sharps (Autodesk Fusion 360 design; units mm, degrees)
Autodesk Fusion 360 part; units mm, degrees
(part 1 of 2)
sketch "Sketch1" plane through (0, 0, 0) normal (0, 1, 0) x (1, 0, 0)
  line L0 (0, 0) -> (-92, 0)
  line L1 (-92, 0) -> (-92, -56)
  line L2 (-92, -56) -> (0, -56)
  line L3 (0, -56) -> (0, 0)
  dimension "d1" = 92
  dimension "d2" = 56
  constraint horizontal L0
  constraint vertical L1
  constraint horizontal L2
  constraint vertical L3
  constraint coincident L0.start L3.end
  measures "d1" distance of L1.end L2.end
  measures "d2" distance of L0.start L2.end
extrude "Extrude1" add sketch "Sketch1" along normal blind 65
shell "Shell1" thickness 3.5 removed faces 1 at (-30.6667, 65, 18.6667)
fillet "Fillet1" radius 5 8 edges at (0, 32.5, 0) (0, 32.5, 56) (-92, 32.5, 56) (-92, 32.5, 0) (-3.5, 34.25, 3.5) (-3.5, 34.25, 52.5) (-88.5, 34.25, 52.5) (-88.5, 34.25, 3.5)
extrude "Extrude2" add 1 faces at (-32.3333, 0, 37.3333) along direction (0, 1, 0) blind 3.5 from surface at 65
sketch "Sketch2" plane through (0, 68.5, 0) normal (0, 1, 0) x (-1, 0, 0)
  line L0 (5, 0) -> (87, 0)
  arc A0 (87, 0) -> (92, 5) centre (87, 5) ccw
  line L1 (92, 5) -> (92, 51)
  arc A1 (92, 51) -> (87, 56) centre (87, 51) ccw
  line L2 (87, 56) -> (5, 56)
  arc A2 (5, 56) -> (0, 51) centre (5, 51) ccw
  line L3 (0, 51) -> (0, 5)
  arc A3 (0, 5) -> (5, 0) centre (5, 5) ccw
  line L4 (85, 26.75) -> (7, 26.75)
  line L5 (7, 26.75) -> (7, 29.25)
  line L6 (7, 29.25) -> (85, 29.25)
  line L7 (85, 29.25) -> (85, 26.75)
  dimension "d11" = 26.75
  dimension "d12" = 26.75
  dimension "d13" = 7
  dimension "d14" = 7
  constraint horizontal L4
  constraint vertical L5
  constraint horizontal L6
  constraint vertical L7
  measures "d11" distance of L0 L4
  measures "d12" distance of L2 L6
  measures "d13" distance of L3 L5
  measures "d14" distance of L1 L7
extrude "Extrude3" cut sketch "Sketch2" against normal blind 40 contours L4 L5 L6 L7
chamfer "Chamfer1" distance 2 angle 45 2 edges at (-46, 68.5, 26.75) (-46, 68.5, 29.25)
ref_plane "WorkPlane1" through (-46, 42.5, 28) normal (0, 1, 0) x (0, 0, 1)
sketch "Sketch3" plane through (0, 65, 0) normal (0, -1, 0) x (1, 0, 0)
  line L0 (-7, 29.25) -> (-7, 26.75)
  line L1 (-7, 26.75) -> (-85, 26.75)
  line L2 (-85, 26.75) -> (-85, 29.25)
  line L3 (-85, 29.25) -> (-7, 29.25)
  arc A0 (-83.5, 52.5) -> (-88.5, 47.5) centre (-83.5, 47.5) ccw
  line L4 (-88.5, 47.5) -> (-88.5, 8.5)
  arc A1 (-88.5, 8.5) -> (-83.5, 3.5) centre (-83.5, 8.5) ccw
  line L5 (-83.5, 3.5) -> (-8.5, 3.5)
  arc A2 (-8.5, 3.5) -> (-3.5, 8.5) centre (-8.5, 8.5) ccw
  line L6 (-3.5, 8.5) -> (-3.5, 47.5)
  arc A3 (-3.5, 47.5) -> (-8.5, 52.5) centre (-8.5, 47.5) ccw
  line L7 (-8.5, 52.5) -> (-83.5, 52.5)
  line L8 (-3.5, 37.1108) -> (-18.952, 52.5)
  line L9 (-73, 52.5) -> (-88.5, 33.8548)
  line L10 (-88.5, 16) -> (-69.7967, 3.5)
  line L11 (-23, 3.5) -> (-3.5, 18.2423)
  line L12 (-3.5, 28) -> (-46, 3.5)
  line L13 (-88.5, 28) -> (-46, 3.5)
  line L14 (-88.5, 28) -> (-46, 52.5)
  line L15 (-3.5, 28) -> (-46, 52.5)
  line L16 (-24.75, 40.25) -> (-67.25, 40.25)
  line L17 (-67.25, 15.75) -> (-24.75, 15.75)
  line L18 (-85, 26.75) -> (-85, 25.9)
  line L19 (-85, 25.9) -> (-85, 30.1)
  line L20 (-7, 26.75) -> (-7, 25.8)
  line L21 (-7, 25.8) -> (-7, 30.2)
  line L22 (-85, 29.25) -> (-46, 40.25)
  line L23 (-7, 29.25) -> (-46, 40.25)
  line L24 (-85, 26.75) -> (-46, 15.75)
  line L25 (-46, 15.75) -> (-7, 26.75)
  line L26 (-26.5, 21.25) -> (-65.5, 21.25)
  line L27 (-65.5, 34.75) -> (-26.5, 34.75)
  constraint coincident L6 L8.start
  constraint coincident L7 L8.end
  constraint coincident L7 L9.start
  constraint coincident L4 L9.end
  constraint coincident L4 L10.start
  constraint coincident L5 L10.end
  constraint coincident L5 L11.start
  constraint coincident L6 L11.end
  constraint midpoint L6 L12.start
  constraint coincident L5 L12.end
  constraint midpoint L4 L13.start
  constraint midpoint L7 L14.end
  constraint midpoint L5 L12.end
  constraint midpoint L15 L16.start
  constraint midpoint L14 L16.end
  constraint midpoint L13 L17.start
  constraint midpoint L12 L17.end
  constraint coincident L1.end L2.start
  constraint perpendicular L1 L18
  constraint parallel L2 L19
  constraint coincident L0.end L1.start
  constraint perpendicular L1 L20
  constraint perpendicular L3 L21
  constraint coincident L2.end L3.start
  constraint midpoint L16 L22.end
  constraint coincident L0.start L3.end
  constraint midpoint L17 L24.end
  constraint midpoint L25 L26.start
  constraint midpoint L24 L26.end
  constraint midpoint L22 L27.start
  constraint midpoint L23 L27.end
sketch "Sketch4" plane through (0, 68.5, 0) normal (0, 1, 0) x (-1, 0, 0)
  line L0 (85, 31.25) -> (85, 24.75)
  line L1 (85, 24.75) -> (7, 24.75)
  line L2 (7, 24.75) -> (7, 31.25)
  line L3 (7, 31.25) -> (85, 31.25)
  line L4 (5, 0) -> (87, 0)
  arc A0 (87, 0) -> (92, 5) centre (87, 5) ccw
  line L5 (92, 5) -> (92, 51)
  arc A1 (92, 51) -> (87, 56) centre (87, 51) ccw
  line L6 (87, 56) -> (5, 56)
  arc A2 (5, 56) -> (0, 51) centre (5, 51) ccw
  line L7 (0, 51) -> (0, 5)
  arc A3 (0, 5) -> (5, 0) centre (5, 5) ccw
  spline S0 degree 3 poles (69.4034, 34.4959) (69.5108, 34.5366) (69.6516, 34.6404) (69.8145, 34.7996) knots 0 0 0 0 1 1 1 1
  spline S1 degree 3 poles (69.8145, 34.7996) (70.0442, 35.0293) (70.3331, 35.522) (74.9596, 43.5267) knots 0 0 0 0 1 1 1 1
  spline S2 degree 3 poles (74.9596, 43.5267) (77.6563, 48.1902) (79.901, 52.0981) (79.9491, 52.2129) knots 0 0 0 0 1 1 1 1
  spline S3 degree 3 poles (79.9491, 52.2129) (80.0492, 52.4574) (80.0603, 52.8241) (79.9751, 53.0723) knots 0 0 0 0 1 1 1 1
  spline S4 degree 3 poles (79.9751, 53.0723) (79.901, 53.2945) (79.7158, 53.5057) (79.4824, 53.6316) knots 0 0 0 0 1 1 1 1
  spline S5 degree 3 poles (79.4824, 53.6316) (79.0787, 53.8539) (79.6861, 53.8428) (68.9552, 53.8428) knots 0 0 0 0 1 1 1 1
  spline S6 degree 3 poles (68.9552, 53.8428) (62.4988, 53.8428) (59.0465, 53.8316) (58.9206, 53.8057) knots 0 0 0 0 1 1 1 1
  spline S7 degree 3 poles (58.9206, 53.8057) (58.4835, 53.7242) (58.139, 53.476) (57.9797, 53.139) knots 0 0 0 0 1 1 1 1
  spline S8 degree 3 poles (57.9797, 53.139) (57.8797, 52.9204) (57.8797, 52.5278) (57.9834, 52.2685) knots 0 0 0 0 1 1 1 1
  spline S9 degree 3 poles (57.9834, 52.2685) (58.0205, 52.1648) (60.2874, 48.2384) (63.0174, 43.5452) knots 0 0 0 0 1 1 1 1
  spline S10 degree 3 poles (63.0174, 43.5452) (68.4477, 34.1959) (68.1514, 34.6774) (68.5996, 34.5107) knots 0 0 0 0 1 1 1 1
  spline S11 degree 3 poles (68.5996, 34.5107) (68.8515, 34.4181) (69.1626, 34.4144) (69.4034, 34.4959) knots 0 0 0 0 1 1 1 1
  spline S12 degree 3 poles (68.6144, 34.6885) (68.5292, 34.7256) (68.3847, 34.833) (68.2921, 34.9256) knots 0 0 0 0 1 1 1 1
  spline S13 degree 3 poles (68.2921, 34.9256) (68.1736, 35.0515) (66.7697, 37.437) (63.1693, 43.6267) knots 0 0 0 0 1 1 1 1
  spline S14 degree 3 poles (63.1693, 43.6267) (60.443, 48.3198) (58.1761, 52.2463) (58.139, 52.3574) knots 0 0 0 0 1 1 1 1
  spline S15 degree 3 poles (58.139, 52.3574) (57.9538, 52.8908) (58.1909, 53.3909) (58.7169, 53.5724) knots 0 0 0 0 1 1 1 1
  spline S16 degree 3 poles (58.7169, 53.5724) (58.891, 53.6353) (59.4577, 53.639) (68.9589, 53.639) knots 0 0 0 0 1 1 1 1
  spline S17 degree 3 poles (68.9589, 53.639) (78.5119, 53.639) (79.0268, 53.6353) (79.2046, 53.5724) knots 0 0 0 0 1 1 1 1
  spline S18 degree 3 poles (79.2046, 53.5724) (79.438, 53.4909) (79.6787, 53.2908) (79.7825, 53.0871) knots 0 0 0 0 1 1 1 1
  spline S19 degree 3 poles (79.7825, 53.0871) (79.8825, 52.8982) (79.8899, 52.4907) (79.7936, 52.2722) knots 0 0 0 0 1 1 1 1
  spline S20 degree 3 poles (79.7936, 52.2722) (79.6824, 52.0129) (69.9183, 35.1589) (69.7849, 34.9997) knots 0 0 0 0 1 1 1 1
  spline S21 degree 3 poles (69.7849, 34.9997) (69.6479, 34.8293) (69.396, 34.6626) (69.2071, 34.6144) knots 0 0 0 0 1 1 1 1
  spline S22 degree 3 poles (69.2071, 34.6144) (69.0515, 34.5774) (68.8033, 34.607) (68.6144, 34.6885) knots 0 0 0 0 1 1 1 1
  spline S23 degree 3 poles (69.2367, 35.2071) (69.3182, 35.2441) (69.4219, 35.3145) (69.4664, 35.3627) knots 0 0 0 0 1 1 1 1
  spline S24 degree 3 poles (69.4664, 35.3627) (69.6034, 35.5145) (79.2528, 52.2166) (79.2787, 52.3463) knots 0 0 0 0 1 1 1 1
  spline S25 degree 3 poles (79.2787, 52.3463) (79.3305, 52.6315) (79.2157, 52.8575) (78.949, 53.0019) knots 0 0 0 0 1 1 1 1
  line L8 (78.949, 53.0019) -> (78.7934, 53.0834)
  line L9 (78.7934, 53.0834) -> (68.9996, 53.0945)
  line L10 (68.9996, 53.0945) -> (59.2058, 53.1019)
  line L11 (59.2058, 53.1019) -> (59.0095, 53.013)
  spline S26 degree 3 poles (59.0095, 53.013) (58.8798, 52.9538) (58.7835, 52.8797) (58.7354, 52.7982) knots 0 0 0 0 1 1 1 1
  spline S27 degree 3 poles (58.7354, 52.7982) (58.6502, 52.6537) (58.6391, 52.413) (58.7132, 52.2389) knots 0 0 0 0 1 1 1 1
  spline S28 degree 3 poles (58.7132, 52.2389) (58.7391, 52.1722) (60.932, 48.3865) (63.5841, 43.823) knots 0 0 0 0 1 1 1 1
  spline S29 degree 3 poles (63.5841, 43.823) (66.7808, 38.326) (68.4588, 35.4738) (68.5588, 35.3738) knots 0 0 0 0 1 1 1 1
  spline S30 degree 3 poles (68.5588, 35.3738) (68.6885, 35.2367) (68.8959, 35.1367) (69.0367, 35.1367) knots 0 0 0 0 1 1 1 1
  spline S31 degree 3 poles (69.0367, 35.1367) (69.0663, 35.1367) (69.1552, 35.1701) (69.2367, 35.2071) knots 0 0 0 0 1 1 1 1
  spline S32 degree 3 poles (64.2398, 44.3156) (61.6802, 48.6643) (59.5873, 52.224) (59.5873, 52.2352) knots 0 0 0 0 1 1 1 1
  spline S33 degree 3 poles (59.5873, 52.2352) (59.5873, 52.2426) (63.8027, 52.25) (68.9589, 52.25) knots 0 0 0 0 1 1 1 1
  spline S34 degree 3 poles (68.9589, 52.25) (74.1151, 52.25) (78.3304, 52.2389) (78.3304, 52.2277) knots 0 0 0 0 1 1 1 1
  spline S35 degree 3 poles (78.3304, 52.2277) (78.3304, 52.1685) (68.9404, 36.3628) (68.9181, 36.3887) knots 0 0 0 0 1 1 1 1
  spline S36 degree 3 poles (68.9181, 36.3887) (68.907, 36.4035) (66.7994, 39.9707) (64.2398, 44.3156) knots 0 0 0 0 1 1 1 1
  spline S37 degree 3 poles (70.0627, 42.6562) (70.9517, 42.7969) (71.4777, 42.8932) (71.537, 42.934) knots 0 0 0 0 1 1 1 1
  spline S38 degree 3 poles (71.537, 42.934) (71.5851, 42.9673) (71.674, 43.0785) (71.7296, 43.1822) knots 0 0 0 0 1 1 1 1
  spline S39 degree 3 poles (71.7296, 43.1822) (71.7852, 43.2896) (71.8741, 43.4229) (71.9296, 43.4785) knots 0 0 0 0 1 1 1 1
  spline S40 degree 3 poles (71.9296, 43.4785) (72.0222, 43.5785) (72.0445, 43.5822) (72.363, 43.5822) knots 0 0 0 0 1 1 1 1
  line L12 (72.363, 43.5822) -> (72.7001, 43.5822)
  line L13 (72.7001, 43.5822) -> (72.7001, 44.6194)
  line L14 (72.7001, 44.6194) -> (72.7001, 45.6566)
  line L15 (72.7001, 45.6566) -> (72.3371, 45.6566)
  spline S41 degree 3 poles (72.3371, 45.6566) (71.9333, 45.6566) (71.9185, 45.664) (71.7407, 45.9603) knots 0 0 0 0 1 1 1 1
  spline S42 degree 3 poles (71.7407, 45.9603) (71.6889, 46.0455) (71.6148, 46.1122) (71.5407, 46.1344) knots 0 0 0 0 1 1 1 1
  spline S43 degree 3 poles (71.5407, 46.1344) (71.337, 46.2011) (68.2921, 46.2048) (67.818, 46.1381) knots 0 0 0 0 1 1 1 1
  spline S44 degree 3 poles (67.818, 46.1381) (67.6698, 46.1196) (67.2031, 46.1011) (66.7882, 46.1011) knots 0 0 0 0 1 1 1 1
  spline S45 degree 3 poles (66.7882, 46.1011) (66.3549, 46.1011) (65.9993, 46.0862) (65.9585, 46.064) knots 0 0 0 0 1 1 1 1
  spline S46 degree 3 poles (65.9585, 46.064) (65.8511, 46.0084) (65.7955, 45.7936) (65.8474, 45.6417) knots 0 0 0 0 1 1 1 1
  spline S47 degree 3 poles (65.8474, 45.6417) (65.9178, 45.4232) (65.9178, 45.4232) (66.7216, 45.4676) knots 0 0 0 0 1 1 1 1
  spline S48 degree 3 poles (66.7216, 45.4676) (67.3846, 45.5047) (67.5217, 45.501) (67.4735, 45.4565) knots 0 0 0 0 1 1 1 1
  spline S49 degree 3 poles (67.4735, 45.4565) (67.4661, 45.4491) (67.0031, 45.4269) (66.4438, 45.4047) knots 0 0 0 0 1 1 1 1
  spline S50 degree 3 poles (66.4438, 45.4047) (65.4584, 45.3713) (65.4251, 45.3676) (65.3584, 45.2861) knots 0 0 0 0 1 1 1 1
  spline S51 degree 3 poles (65.3584, 45.2861) (65.2732, 45.1824) (65.2695, 44.9268) (65.351, 44.8083) knots 0 0 0 0 1 1 1 1
  line L16 (65.351, 44.8083) -> (65.414, 44.7194)
  line L17 (65.414, 44.7194) -> (66.3808, 44.7416)
  spline S52 degree 3 poles (66.3808, 44.7416) (66.9623, 44.7527) (67.2068, 44.749) (66.9957, 44.7305) knots 0 0 0 0 1 1 1 1
  spline S53 degree 3 poles (66.9957, 44.7305) (66.8031, 44.7157) (66.2622, 44.7009) (65.7992, 44.6972) knots 0 0 0 0 1 1 1 1
  line L18 (65.7992, 44.6972) -> (64.9547, 44.6935)
  line L19 (64.9547, 44.6935) -> (64.8658, 44.6009)
  spline S54 degree 3 poles (64.8658, 44.6009) (64.7547, 44.4934) (64.7398, 44.2416) (64.8361, 44.1045) knots 0 0 0 0 1 1 1 1
  line L20 (64.8361, 44.1045) -> (64.8954, 44.0156)
  line L21 (64.8954, 44.0156) -> (66.04, 44.0415)
  spline S55 degree 3 poles (66.04, 44.0415) (66.7253, 44.0564) (67.1809, 44.0526) (67.1809, 44.0341) knots 0 0 0 0 1 1 1 1
  spline S56 degree 3 poles (67.1809, 44.0341) (67.1809, 43.9934) (66.8549, 43.9637) (66.0363, 43.9304) knots 0 0 0 0 1 1 1 1
  spline S57 degree 3 poles (66.0363, 43.9304) (65.3658, 43.9008) (65.3288, 43.8823) (65.3288, 43.5896) knots 0 0 0 0 1 1 1 1
  spline S58 degree 3 poles (65.3288, 43.5896) (65.3288, 43.4933) (65.3547, 43.3785) (65.3807, 43.3377) knots 0 0 0 0 1 1 1 1
  spline S59 degree 3 poles (65.3807, 43.3377) (65.4362, 43.2637) (65.4621, 43.26) (67.0586, 43.2563) knots 0 0 0 0 1 1 1 1
  spline S60 degree 3 poles (67.0586, 43.2563) (67.9921, 43.2525) (68.8589, 43.2674) (69.0996, 43.2896) knots 0 0 0 0 1 1 1 1
  spline S61 degree 3 poles (69.0996, 43.2896) (69.3293, 43.3118) (69.5256, 43.3229) (69.5367, 43.3155) knots 0 0 0 0 1 1 1 1
  spline S62 degree 3 poles (69.5367, 43.3155) (69.5441, 43.3044) (69.3886, 43.2525) (69.1922, 43.1933) knots 0 0 0 0 1 1 1 1
  spline S63 degree 3 poles (69.1922, 43.1933) (68.7774, 43.0785) (68.67, 43.0007) (68.5514, 42.7229) knots 0 0 0 0 1 1 1 1
  spline S64 degree 3 poles (68.5514, 42.7229) (68.4625, 42.5117) (68.4736, 42.4339) (68.5959, 42.4376) knots 0 0 0 0 1 1 1 1
  spline S65 degree 3 poles (68.5959, 42.4376) (68.644, 42.4413) (69.3034, 42.5376) (70.0627, 42.6562) knots 0 0 0 0 1 1 1 1
  spline S66 degree 3 poles (68.6625, 43.4229) (68.6588, 43.4415) (68.7885, 43.8971) (68.9478, 44.4416) knots 0 0 0 0 1 1 1 1
  line L22 (68.9478, 44.4416) -> (69.2367, 45.4306)
  line L23 (69.2367, 45.4306) -> (69.2478, 44.4638)
  spline S67 degree 3 poles (69.2478, 44.4638) (69.2515, 43.9304) (69.2478, 43.4896) (69.2367, 43.4785) knots 0 0 0 0 1 1 1 1
  spline S68 degree 3 poles (69.2367, 43.4785) (69.2256, 43.4674) (69.107, 43.4452) (68.9663, 43.4341) knots 0 0 0 0 1 1 1 1
  spline S69 degree 3 poles (68.9663, 43.4341) (68.8292, 43.4192) (68.707, 43.4044) (68.6885, 43.4007) knots 0 0 0 0 1 1 1 1
  spline S70 degree 3 poles (68.6885, 43.4007) (68.6737, 43.4007) (68.6625, 43.4081) (68.6625, 43.4229) knots 0 0 0 0 1 1 1 1
  spline S71 degree 3 poles (67.8476, 43.4303) (67.8476, 43.4452) (67.9884, 43.9008) (68.1625, 44.4379) knots 0 0 0 0 1 1 1 1
  line L24 (68.1625, 44.4379) -> (68.4736, 45.4158)
  line L25 (68.4736, 45.4158) -> (68.4736, 44.9342)
  spline S72 degree 3 poles (68.4736, 44.9342) (68.4773, 44.6675) (68.4662, 44.2156) (68.4514, 43.923) knots 0 0 0 0 1 1 1 1
  line L26 (68.4514, 43.923) -> (68.4292, 43.397)
  line L27 (68.4292, 43.397) -> (68.1366, 43.397)
  spline S73 degree 3 poles (68.1366, 43.397) (67.9773, 43.397) (67.8476, 43.4118) (67.8476, 43.4303) knots 0 0 0 0 1 1 1 1
  spline S74 degree 3 poles (67.3253, 43.4341) (67.2253, 43.4341) (67.2327, 43.6637) (67.3476, 44.2045) knots 0 0 0 0 1 1 1 1
  spline S75 degree 3 poles (67.3476, 44.2045) (67.4735, 44.7898) (67.7735, 45.927) (67.8143, 45.9677) knots 0 0 0 0 1 1 1 1
  spline S76 degree 3 poles (67.8143, 45.9677) (67.8587, 46.0159) (67.8624, 46.0529) (67.755, 44.7676) knots 0 0 0 0 1 1 1 1
  spline S77 degree 3 poles (67.755, 44.7676) (67.6328, 43.2933) (67.6476, 43.3822) (67.5068, 43.4118) knots 0 0 0 0 1 1 1 1
  spline S78 degree 3 poles (67.5068, 43.4118) (67.4439, 43.4229) (67.3624, 43.4341) (67.3253, 43.4341) knots 0 0 0 0 1 1 1 1
  line L28 (69.4404, 44.8972) -> (69.4404, 46.027)
  line L29 (69.4404, 46.027) -> (69.7368, 46.027)
  spline S79 degree 3 poles (69.7368, 46.027) (69.9664, 46.027) (70.0331, 46.0159) (70.0331, 45.9751) knots 0 0 0 0 1 1 1 1
  spline S80 degree 3 poles (70.0331, 45.9751) (70.0331, 45.7269) (69.5219, 43.7674) (69.4589, 43.7674) knots 0 0 0 0 1 1 1 1
  spline S81 degree 3 poles (69.4589, 43.7674) (69.4478, 43.7674) (69.4404, 44.2749) (69.4404, 44.8972) knots 0 0 0 0 1 1 1 1
  line L30 (68.6514, 45.038) -> (68.6737, 46.027)
  line L31 (68.6737, 46.027) -> (68.9478, 46.027)
  spline S82 degree 3 poles (68.9478, 46.027) (69.0959, 46.027) (69.2182, 46.0159) (69.2182, 45.9973) knots 0 0 0 0 1 1 1 1
  spline S83 degree 3 poles (69.2182, 45.9973) (69.2219, 45.9529) (68.6477, 44.0304) (68.6366, 44.0415) knots 0 0 0 0 1 1 1 1
  spline S84 degree 3 poles (68.6366, 44.0415) (68.6292, 44.0452) (68.6366, 44.4971) (68.6514, 45.038) knots 0 0 0 0 1 1 1 1
  spline S85 degree 3 poles (67.9513, 45.1528) (68.0032, 45.7455) (68.0365, 45.9677) (68.0736, 45.9936) knots 0 0 0 0 1 1 1 1
  spline S86 degree 3 poles (68.0736, 45.9936) (68.1588, 46.0455) (68.4885, 46.0344) (68.4699, 45.9788) knots 0 0 0 0 1 1 1 1
  spline S87 degree 3 poles (68.4699, 45.9788) (68.4588, 45.9566) (68.3292, 45.5417) (68.1773, 45.0565) knots 0 0 0 0 1 1 1 1
  spline S88 degree 3 poles (68.1773, 45.0565) (68.0254, 44.5749) (67.8995, 44.2156) (67.8921, 44.2601) knots 0 0 0 0 1 1 1 1
  spline S89 degree 3 poles (67.8921, 44.2601) (67.8884, 44.3045) (67.9143, 44.7046) (67.9513, 45.1528) knots 0 0 0 0 1 1 1 1
  line L32 (69.3071, 47.9568) -> (70.1442, 49.031)
  line L33 (70.1442, 49.031) -> (70.1442, 50.4942)
  line L34 (70.1442, 50.4942) -> (70.1442, 51.9536)
  line L35 (70.1442, 51.9536) -> (69.2923, 51.9536)
  line L36 (69.2923, 51.9536) -> (68.4403, 51.9536)
  line L37 (68.4403, 51.9536) -> (68.4403, 49.4163)
  spline S90 degree 3 poles (68.4403, 49.4163) (68.4403, 48.0198) (68.4477, 46.8789) (68.4551, 46.8789) knots 0 0 0 0 1 1 1 1
  spline S91 degree 3 poles (68.4551, 46.8789) (68.4662, 46.8789) (68.8478, 47.3642) (69.3071, 47.9568) knots 0 0 0 0 1 1 1 1
  spline S92 degree 3 poles (57.9797, 53.139) (57.8797, 52.9204) (57.8797, 52.5278) (57.9834, 52.2685) knots 0 0 0 0 1 1 1 1
  line L38 (69.2923, 51.9536) -> (68.4403, 51.9536)
  spline S93 degree 3 poles (64.2398, 44.3156) (61.6802, 48.6643) (59.5873, 52.224) (59.5873, 52.2352) knots 0 0 0 0 1 1 1 1
  line L39 (68.4403, 51.9536) -> (68.4403, 49.4163)
  spline S94 degree 3 poles (57.9834, 52.2685) (58.0205, 52.1648) (60.2874, 48.2384) (63.0174, 43.5452) knots 0 0 0 0 1 1 1 1
  spline S95 degree 3 poles (59.0095, 53.013) (58.8798, 52.9538) (58.7835, 52.8797) (58.7354, 52.7982) knots 0 0 0 0 1 1 1 1
  spline S96 degree 3 poles (58.139, 52.3574) (57.9538, 52.8908) (58.1909, 53.3909) (58.7169, 53.5724) knots 0 0 0 0 1 1 1 1
  spline S97 degree 3 poles (69.5367, 43.3155) (69.5441, 43.3044) (69.3886, 43.2525) (69.1922, 43.1933) knots 0 0 0 0 1 1 1 1
  spline S98 degree 3 poles (67.4735, 45.4565) (67.4661, 45.4491) (67.0031, 45.4269) (66.4438, 45.4047) knots 0 0 0 0 1 1 1 1
  spline S99 degree 3 poles (67.8921, 44.2601) (67.8884, 44.3045) (67.9143, 44.7046) (67.9513, 45.1528) knots 0 0 0 0 1 1 1 1
  spline S100 degree 3 poles (68.5959, 42.4376) (68.644, 42.4413) (69.3034, 42.5376) (70.0627, 42.6562) knots 0 0 0 0 1 1 1 1
  line L40 (65.414, 44.7194) -> (66.3808, 44.7416)
  line L41 (69.3071, 47.9568) -> (70.1442, 49.031)
  spline S101 degree 3 poles (65.8474, 45.6417) (65.9178, 45.4232) (65.9178, 45.4232) (66.7216, 45.4676) knots 0 0 0 0 1 1 1 1
  line L42 (70.1442, 49.031) -> (70.1442, 50.4942)
  spline S102 degree 3 poles (67.1809, 44.0341) (67.1809, 43.9934) (66.8549, 43.9637) (66.0363, 43.9304) knots 0 0 0 0 1 1 1 1
  line L43 (70.1442, 51.9536) -> (69.2923, 51.9536)
  spline S103 degree 3 poles (70.0627, 42.6562) (70.9517, 42.7969) (71.4777, 42.8932) (71.537, 42.934) knots 0 0 0 0 1 1 1 1
  spline S104 degree 3 poles (64.8658, 44.6009) (64.7547, 44.4934) (64.7398, 44.2416) (64.8361, 44.1045) knots 0 0 0 0 1 1 1 1
  line L44 (72.7001, 43.5822) -> (72.7001, 44.6194)
  spline S105 degree 3 poles (66.9957, 44.7305) (66.8031, 44.7157) (66.2622, 44.7009) (65.7992, 44.6972) knots 0 0 0 0 1 1 1 1
  line L45 (68.4292, 43.397) -> (68.1366, 43.397)
  spline S106 degree 3 poles (69.2182, 45.9973) (69.2219, 45.9529) (68.6477, 44.0304) (68.6366, 44.0415) knots 0 0 0 0 1 1 1 1
  spline S107 degree 3 poles (67.8476, 43.4303) (67.8476, 43.4452) (67.9884, 43.9008) (68.1625, 44.4379) knots 0 0 0 0 1 1 1 1
  line L46 (68.4736, 45.4158) -> (68.4736, 44.9342)
  spline S108 degree 3 poles (66.04, 44.0415) (66.7253, 44.0564) (67.1809, 44.0526) (67.1809, 44.0341) knots 0 0 0 0 1 1 1 1
  spline S109 degree 3 poles (69.4589, 43.7674) (69.4478, 43.7674) (69.4404, 44.2749) (69.4404, 44.8972) knots 0 0 0 0 1 1 1 1
  spline S110 degree 3 poles (68.5514, 42.7229) (68.4625, 42.5117) (68.4736, 42.4339) (68.5959, 42.4376) knots 0 0 0 0 1 1 1 1
  spline S111 degree 3 poles (68.4699, 45.9788) (68.4588, 45.9566) (68.3292, 45.5417) (68.1773, 45.0565) knots 0 0 0 0 1 1 1 1
  spline S112 degree 3 poles (67.3476, 44.2045) (67.4735, 44.7898) (67.7735, 45.927) (67.8143, 45.9677) knots 0 0 0 0 1 1 1 1
  line L47 (64.9547, 44.6935) -> (64.8658, 44.6009)
  spline S113 degree 3 poles (71.9296, 43.4785) (72.0222, 43.5785) (72.0445, 43.5822) (72.363, 43.5822) knots 0 0 0 0 1 1 1 1
  spline S114 degree 3 poles (65.3584, 45.2861) (65.2732, 45.1824) (65.2695, 44.9268) (65.351, 44.8083) knots 0 0 0 0 1 1 1 1
  line L48 (64.8361, 44.1045) -> (64.8954, 44.0156)
  spline S115 degree 3 poles (69.1922, 43.1933) (68.7774, 43.0785) (68.67, 43.0007) (68.5514, 42.7229) knots 0 0 0 0 1 1 1 1
  spline S116 degree 3 poles (68.4403, 49.4163) (68.4403, 48.0198) (68.4477, 46.8789) (68.4551, 46.8789) knots 0 0 0 0 1 1 1 1
  line L49 (59.2058, 53.1019) -> (59.0095, 53.013)
  spline S117 degree 3 poles (68.9589, 52.25) (74.1151, 52.25) (78.3304, 52.2389) (78.3304, 52.2277) knots 0 0 0 0 1 1 1 1
  spline S118 degree 3 poles (68.4551, 46.8789) (68.4662, 46.8789) (68.8478, 47.3642) (69.3071, 47.9568) knots 0 0 0 0 1 1 1 1
  line L50 (68.9996, 53.0945) -> (59.2058, 53.1019)
  spline S119 degree 3 poles (68.1366, 43.397) (67.9773, 43.397) (67.8476, 43.4118) (67.8476, 43.4303) knots 0 0 0 0 1 1 1 1
  spline S120 degree 3 poles (59.5873, 52.2352) (59.5873, 52.2426) (63.8027, 52.25) (68.9589, 52.25) knots 0 0 0 0 1 1 1 1
  spline S121 degree 3 poles (67.0586, 43.2563) (67.9921, 43.2525) (68.8589, 43.2674) (69.0996, 43.2896) knots 0 0 0 0 1 1 1 1
  spline S122 degree 3 poles (65.3288, 43.5896) (65.3288, 43.4933) (65.3547, 43.3785) (65.3807, 43.3377) knots 0 0 0 0 1 1 1 1
  line L51 (68.4514, 43.923) -> (68.4292, 43.397)
  spline S123 degree 3 poles (71.537, 42.934) (71.5851, 42.9673) (71.674, 43.0785) (71.7296, 43.1822) knots 0 0 0 0 1 1 1 1
  line L52 (78.949, 53.0019) -> (78.7934, 53.0834)
  spline S124 degree 3 poles (69.0367, 35.1367) (69.0663, 35.1367) (69.1552, 35.1701) (69.2367, 35.2071) knots 0 0 0 0 1 1 1 1
  spline S125 degree 3 poles (69.2367, 35.2071) (69.3182, 35.2441) (69.4219, 35.3145) (69.4664, 35.3627) knots 0 0 0 0 1 1 1 1
  spline S126 degree 3 poles (68.9552, 53.8428) (62.4988, 53.8428) (59.0465, 53.8316) (58.9206, 53.8057) knots 0 0 0 0 1 1 1 1
  spline S127 degree 3 poles (69.4664, 35.3627) (69.6034, 35.5145) (79.2528, 52.2166) (79.2787, 52.3463) knots 0 0 0 0 1 1 1 1
  spline S128 degree 3 poles (79.7936, 52.2722) (79.6824, 52.0129) (69.9183, 35.1589) (69.7849, 34.9997) knots 0 0 0 0 1 1 1 1
  spline S129 degree 3 poles (78.3304, 52.2277) (78.3304, 52.1685) (68.9404, 36.3628) (68.9181, 36.3887) knots 0 0 0 0 1 1 1 1
  spline S130 degree 3 poles (69.8145, 34.7996) (70.0442, 35.0293) (70.3331, 35.522) (74.9596, 43.5267) knots 0 0 0 0 1 1 1 1
  spline S131 degree 3 poles (68.9589, 53.639) (78.5119, 53.639) (79.0268, 53.6353) (79.2046, 53.5724) knots 0 0 0 0 1 1 1 1
  spline S132 degree 3 poles (79.4824, 53.6316) (79.0787, 53.8539) (79.6861, 53.8428) (68.9552, 53.8428) knots 0 0 0 0 1 1 1 1
  spline S133 degree 3 poles (63.5841, 43.823) (66.7808, 38.326) (68.4588, 35.4738) (68.5588, 35.3738) knots 0 0 0 0 1 1 1 1
  spline S134 degree 3 poles (58.7169, 53.5724) (58.891, 53.6353) (59.4577, 53.639) (68.9589, 53.639) knots 0 0 0 0 1 1 1 1
  spline S135 degree 3 poles (68.6144, 34.6885) (68.5292, 34.7256) (68.3847, 34.833) (68.2921, 34.9256) knots 0 0 0 0 1 1 1 1
  spline S136 degree 3 poles (68.9181, 36.3887) (68.907, 36.4035) (66.7994, 39.9707) (64.2398, 44.3156) knots 0 0 0 0 1 1 1 1
  spline S137 degree 3 poles (69.2071, 34.6144) (69.0515, 34.5774) (68.8033, 34.607) (68.6144, 34.6885) knots 0 0 0 0 1 1 1 1
  spline S138 degree 3 poles (68.2921, 34.9256) (68.1736, 35.0515) (66.7697, 37.437) (63.1693, 43.6267) knots 0 0 0 0 1 1 1 1
  spline S139 degree 3 poles (69.2367, 43.4785) (69.2256, 43.4674) (69.107, 43.4452) (68.9663, 43.4341) knots 0 0 0 0 1 1 1 1
  spline S140 degree 3 poles (65.3807, 43.3377) (65.4362, 43.2637) (65.4621, 43.26) (67.0586, 43.2563) knots 0 0 0 0 1 1 1 1
  spline S141 degree 3 poles (66.0363, 43.9304) (65.3658, 43.9008) (65.3288, 43.8823) (65.3288, 43.5896) knots 0 0 0 0 1 1 1 1
  spline S142 degree 3 poles (68.1773, 45.0565) (68.0254, 44.5749) (67.8995, 44.2156) (67.8921, 44.2601) knots 0 0 0 0 1 1 1 1
  spline S143 degree 3 poles (66.4438, 45.4047) (65.4584, 45.3713) (65.4251, 45.3676) (65.3584, 45.2861) knots 0 0 0 0 1 1 1 1
  spline S144 degree 3 poles (66.7216, 45.4676) (67.3846, 45.5047) (67.5217, 45.501) (67.4735, 45.4565) knots 0 0 0 0 1 1 1 1
  line L53 (65.351, 44.8083) -> (65.414, 44.7194)
  line L54 (72.7001, 44.6194) -> (72.7001, 45.6566)
  line L55 (64.8954, 44.0156) -> (66.04, 44.0415)
  spline S145 degree 3 poles (68.6625, 43.4229) (68.6588, 43.4415) (68.7885, 43.8971) (68.9478, 44.4416) knots 0 0 0 0 1 1 1 1
  spline S146 degree 3 poles (71.7407, 45.9603) (71.6889, 46.0455) (71.6148, 46.1122) (71.5407, 46.1344) knots 0 0 0 0 1 1 1 1
  line L56 (68.1625, 44.4379) -> (68.4736, 45.4158)
  spline S147 degree 3 poles (67.3253, 43.4341) (67.2253, 43.4341) (67.2327, 43.6637) (67.3476, 44.2045) knots 0 0 0 0 1 1 1 1
  spline S148 degree 3 poles (65.9585, 46.064) (65.8511, 46.0084) (65.7955, 45.7936) (65.8474, 45.6417) knots 0 0 0 0 1 1 1 1
  line L57 (65.7992, 44.6972) -> (64.9547, 44.6935)
  spline S149 degree 3 poles (68.9663, 43.4341) (68.8292, 43.4192) (68.707, 43.4044) (68.6885, 43.4007) knots 0 0 0 0 1 1 1 1
  spline S150 degree 3 poles (69.7368, 46.027) (69.9664, 46.027) (70.0331, 46.0159) (70.0331, 45.9751) knots 0 0 0 0 1 1 1 1
  spline S151 degree 3 poles (69.0996, 43.2896) (69.3293, 43.3118) (69.5256, 43.3229) (69.5367, 43.3155) knots 0 0 0 0 1 1 1 1
  spline S152 degree 3 poles (67.8143, 45.9677) (67.8587, 46.0159) (67.8624, 46.0529) (67.755, 44.7676) knots 0 0 0 0 1 1 1 1
  spline S153 degree 3 poles (70.0331, 45.9751) (70.0331, 45.7269) (69.5219, 43.7674) (69.4589, 43.7674) knots 0 0 0 0 1 1 1 1
  spline S154 degree 3 poles (68.4736, 44.9342) (68.4773, 44.6675) (68.4662, 44.2156) (68.4514, 43.923) knots 0 0 0 0 1 1 1 1
  spline S155 degree 3 poles (67.755, 44.7676) (67.6328, 43.2933) (67.6476, 43.3822) (67.5068, 43.4118) knots 0 0 0 0 1 1 1 1
  line L58 (68.6737, 46.027) -> (68.9478, 46.027)
  spline S156 degree 3 poles (69.2478, 44.4638) (69.2515, 43.9304) (69.2478, 43.4896) (69.2367, 43.4785) knots 0 0 0 0 1 1 1 1
  line L59 (70.1442, 50.4942) -> (70.1442, 51.9536)
  spline S157 degree 3 poles (66.3808, 44.7416) (66.9623, 44.7527) (67.2068, 44.749) (66.9957, 44.7305) knots 0 0 0 0 1 1 1 1
  spline S158 degree 3 poles (66.7882, 46.1011) (66.3549, 46.1011) (65.9993, 46.0862) (65.9585, 46.064) knots 0 0 0 0 1 1 1 1
  line L60 (72.7001, 45.6566) -> (72.3371, 45.6566)
  spline S159 degree 3 poles (71.7296, 43.1822) (71.7852, 43.2896) (71.8741, 43.4229) (71.9296, 43.4785) knots 0 0 0 0 1 1 1 1
  line L61 (68.9478, 44.4416) -> (69.2367, 45.4306)
  spline S160 degree 3 poles (68.6366, 44.0415) (68.6292, 44.0452) (68.6366, 44.4971) (68.6514, 45.038) knots 0 0 0 0 1 1 1 1
  spline S161 degree 3 poles (68.9478, 46.027) (69.0959, 46.027) (69.2182, 46.0159) (69.2182, 45.9973) knots 0 0 0 0 1 1 1 1
  spline S162 degree 3 poles (68.6885, 43.4007) (68.6737, 43.4007) (68.6625, 43.4081) (68.6625, 43.4229) knots 0 0 0 0 1 1 1 1
  spline S163 degree 3 poles (72.3371, 45.6566) (71.9333, 45.6566) (71.9185, 45.664) (71.7407, 45.9603) knots 0 0 0 0 1 1 1 1
  spline S164 degree 3 poles (71.5407, 46.1344) (71.337, 46.2011) (68.2921, 46.2048) (67.818, 46.1381) knots 0 0 0 0 1 1 1 1
  spline S165 degree 3 poles (67.5068, 43.4118) (67.4439, 43.4229) (67.3624, 43.4341) (67.3253, 43.4341) knots 0 0 0 0 1 1 1 1
  line L62 (69.4404, 46.027) -> (69.7368, 46.027)
  line L63 (68.6514, 45.038) -> (68.6737, 46.027)
  spline S166 degree 3 poles (67.9513, 45.1528) (68.0032, 45.7455) (68.0365, 45.9677) (68.0736, 45.9936) knots 0 0 0 0 1 1 1 1
  line L64 (69.2367, 45.4306) -> (69.2478, 44.4638)
  line L65 (72.363, 43.5822) -> (72.7001, 43.5822)
  line L66 (69.4404, 44.8972) -> (69.4404, 46.027)
  spline S167 degree 3 poles (68.0736, 45.9936) (68.1588, 46.0455) (68.4885, 46.0344) (68.4699, 45.9788) knots 0 0 0 0 1 1 1 1
  spline S168 degree 3 poles (67.818, 46.1381) (67.6698, 46.1196) (67.2031, 46.1011) (66.7882, 46.1011) knots 0 0 0 0 1 1 1 1
  spline S169 degree 3 poles (79.2046, 53.5724) (79.438, 53.4909) (79.6787, 53.2908) (79.7825, 53.0871) knots 0 0 0 0 1 1 1 1
  spline S170 degree 3 poles (79.7825, 53.0871) (79.8825, 52.8982) (79.8899, 52.4907) (79.7936, 52.2722) knots 0 0 0 0 1 1 1 1
  spline S171 degree 3 poles (79.9751, 53.0723) (79.901, 53.2945) (79.7158, 53.5057) (79.4824, 53.6316) knots 0 0 0 0 1 1 1 1
  spline S172 degree 3 poles (74.9596, 43.5267) (77.6563, 48.1902) (79.901, 52.0981) (79.9491, 52.2129) knots 0 0 0 0 1 1 1 1
  spline S173 degree 3 poles (79.2787, 52.3463) (79.3305, 52.6315) (79.2157, 52.8575) (78.949, 53.0019) knots 0 0 0 0 1 1 1 1
  spline S174 degree 3 poles (69.4034, 34.4959) (69.5108, 34.5366) (69.6516, 34.6404) (69.8145, 34.7996) knots 0 0 0 0 1 1 1 1
  spline S175 degree 3 poles (79.9491, 52.2129) (80.0492, 52.4574) (80.0603, 52.8241) (79.9751, 53.0723) knots 0 0 0 0 1 1 1 1
  line L67 (78.7934, 53.0834) -> (68.9996, 53.0945)
  spline S176 degree 3 poles (69.7849, 34.9997) (69.6479, 34.8293) (69.396, 34.6626) (69.2071, 34.6144) knots 0 0 0 0 1 1 1 1
  spline S177 degree 3 poles (68.5996, 34.5107) (68.8515, 34.4181) (69.1626, 34.4144) (69.4034, 34.4959) knots 0 0 0 0 1 1 1 1
  spline S178 degree 3 poles (68.5588, 35.3738) (68.6885, 35.2367) (68.8959, 35.1367) (69.0367, 35.1367) knots 0 0 0 0 1 1 1 1
  spline S179 degree 3 poles (63.0174, 43.5452) (68.4477, 34.1959) (68.1514, 34.6774) (68.5996, 34.5107) knots 0 0 0 0 1 1 1 1
  spline S180 degree 3 poles (58.9206, 53.8057) (58.4835, 53.7242) (58.139, 53.476) (57.9797, 53.139) knots 0 0 0 0 1 1 1 1
  spline S181 degree 3 poles (58.7354, 52.7982) (58.6502, 52.6537) (58.6391, 52.413) (58.7132, 52.2389) knots 0 0 0 0 1 1 1 1
  spline S182 degree 3 poles (63.1693, 43.6267) (60.443, 48.3198) (58.1761, 52.2463) (58.139, 52.3574) knots 0 0 0 0 1 1 1 1
  spline S183 degree 3 poles (58.7132, 52.2389) (58.7391, 52.1722) (60.932, 48.3865) (63.5841, 43.823) knots 0 0 0 0 1 1 1 1
  line L68 (83.5, 3.5, -3.5) -> (8.5, 3.5, -3.5)
  line L69 (8.5, 52.5, -3.5) -> (83.5, 52.5, -3.5)
  line L70 (46, 3.5, -3.5) -> (46, 52.5, -3.5)
  line L71 (46, 0) -> (46, 56)
  spline S184 degree 3 poles (32.4127, 52.2352) (32.4127, 52.2426) (28.1973, 52.25) (23.0411, 52.25) knots 0 0 0 0 1 1 1 1
  spline S185 degree 3 poles (32.4127, 52.2352) (32.4127, 52.2426) (28.1973, 52.25) (23.0411, 52.25) knots 0 0 0 0 1 1 1 1
  spline S186 degree 3 poles (33.2868, 52.2389) (33.2609, 52.1722) (31.068, 48.3865) (28.4159, 43.823) knots 0 0 0 0 1 1 1 1
  line L72 (23.0004, 53.0945) -> (32.7942, 53.1019)
  spline S187 degree 3 poles (23.3634, 44.0415) (23.3708, 44.0452) (23.3634, 44.4971) (23.3486, 45.038) knots 0 0 0 0 1 1 1 1
  spline S188 degree 3 poles (25.96, 44.0415) (25.2747, 44.0564) (24.8191, 44.0526) (24.8191, 44.0341) knots 0 0 0 0 1 1 1 1
  spline S189 degree 3 poles (26.6416, 45.2861) (26.7268, 45.1824) (26.7305, 44.9268) (26.649, 44.8083) knots 0 0 0 0 1 1 1 1
  spline S190 degree 3 poles (25.5562, 45.4047) (26.5416, 45.3713) (26.5749, 45.3676) (26.6416, 45.2861) knots 0 0 0 0 1 1 1 1
  spline S191 degree 3 poles (23.3115, 43.4007) (23.3263, 43.4007) (23.3375, 43.4081) (23.3375, 43.4229) knots 0 0 0 0 1 1 1 1
  spline S192 degree 3 poles (24.1857, 45.9677) (24.1413, 46.0159) (24.1376, 46.0529) (24.245, 44.7676) knots 0 0 0 0 1 1 1 1
  line L73 (27.1639, 44.1045) -> (27.1046, 44.0156)
  spline S193 degree 3 poles (26.6193, 43.3377) (26.5638, 43.2637) (26.5379, 43.26) (24.9414, 43.2563) knots 0 0 0 0 1 1 1 1
  line L74 (23.8375, 44.4379) -> (23.5264, 45.4158)
  spline S194 degree 3 poles (23.5301, 45.9788) (23.5412, 45.9566) (23.6708, 45.5417) (23.8227, 45.0565) knots 0 0 0 0 1 1 1 1
  line L75 (27.1046, 44.0156) -> (25.96, 44.0415)
  spline S195 degree 3 poles (23.3634, 44.0415) (23.3708, 44.0452) (23.3634, 44.4971) (23.3486, 45.038) knots 0 0 0 0 1 1 1 1
  line L76 (23.8375, 44.4379) -> (23.5264, 45.4158)
  spline S196 degree 3 poles (24.1079, 44.2601) (24.1116, 44.3045) (24.0857, 44.7046) (24.0487, 45.1528) knots 0 0 0 0 1 1 1 1
  spline S197 degree 3 poles (23.9264, 45.9936) (23.8412, 46.0455) (23.5115, 46.0344) (23.5301, 45.9788) knots 0 0 0 0 1 1 1 1
  line L77 (23.3263, 46.027) -> (23.0522, 46.027)
  spline S198 degree 3 poles (24.6524, 44.2045) (24.5265, 44.7898) (24.2265, 45.927) (24.1857, 45.9677) knots 0 0 0 0 1 1 1 1
  spline S199 degree 3 poles (23.5301, 45.9788) (23.5412, 45.9566) (23.6708, 45.5417) (23.8227, 45.0565) knots 0 0 0 0 1 1 1 1
  spline S200 degree 3 poles (24.6524, 44.2045) (24.5265, 44.7898) (24.2265, 45.927) (24.1857, 45.9677) knots 0 0 0 0 1 1 1 1
  spline S201 degree 3 poles (23.4486, 42.7229) (23.5375, 42.5117) (23.5264, 42.4339) (23.4041, 42.4376) knots 0 0 0 0 1 1 1 1
  spline S202 degree 3 poles (25.9637, 43.9304) (26.6342, 43.9008) (26.6712, 43.8823) (26.6712, 43.5896) knots 0 0 0 0 1 1 1 1
  spline S203 degree 3 poles (25.6192, 44.7416) (25.0377, 44.7527) (24.7932, 44.749) (25.0043, 44.7305) knots 0 0 0 0 1 1 1 1
  spline S204 degree 3 poles (25.2118, 46.1011) (25.6451, 46.1011) (26.0007, 46.0862) (26.0415, 46.064) knots 0 0 0 0 1 1 1 1
  line L78 (23.5486, 43.923) -> (23.5708, 43.397)
  spline S205 degree 3 poles (23.3115, 43.4007) (23.3263, 43.4007) (23.3375, 43.4081) (23.3375, 43.4229) knots 0 0 0 0 1 1 1 1
  spline S206 degree 3 poles (22.7522, 44.4638) (22.7485, 43.9304) (22.7522, 43.4896) (22.7633, 43.4785) knots 0 0 0 0 1 1 1 1
  line L79 (27.1046, 44.0156) -> (25.96, 44.0415)
  spline S207 degree 3 poles (23.4486, 42.7229) (23.5375, 42.5117) (23.5264, 42.4339) (23.4041, 42.4376) knots 0 0 0 0 1 1 1 1
  spline S208 degree 3 poles (23.8634, 43.397) (24.0227, 43.397) (24.1524, 43.4118) (24.1524, 43.4303) knots 0 0 0 0 1 1 1 1
  spline S209 degree 3 poles (22.7633, 43.4785) (22.7744, 43.4674) (22.893, 43.4452) (23.0337, 43.4341) knots 0 0 0 0 1 1 1 1
  spline S210 degree 3 poles (24.1857, 45.9677) (24.1413, 46.0159) (24.1376, 46.0529) (24.245, 44.7676) knots 0 0 0 0 1 1 1 1
  spline S211 degree 3 poles (26.6712, 43.5896) (26.6712, 43.4933) (26.6453, 43.3785) (26.6193, 43.3377) knots 0 0 0 0 1 1 1 1
  spline S212 degree 3 poles (23.9264, 45.9936) (23.8412, 46.0455) (23.5115, 46.0344) (23.5301, 45.9788) knots 0 0 0 0 1 1 1 1
  line L80 (26.649, 44.8083) -> (26.586, 44.7194)
  line L81 (27.1639, 44.1045) -> (27.1046, 44.0156)
  line L82 (23.5264, 45.4158) -> (23.5264, 44.9342)
  line L83 (23.5486, 43.923) -> (23.5708, 43.397)
  spline S213 degree 3 poles (26.1526, 45.6417) (26.0822, 45.4232) (26.0822, 45.4232) (25.2784, 45.4676) knots 0 0 0 0 1 1 1 1
  spline S214 degree 3 poles (26.0415, 46.064) (26.1489, 46.0084) (26.2045, 45.7936) (26.1526, 45.6417) knots 0 0 0 0 1 1 1 1
  line L84 (26.586, 44.7194) -> (25.6192, 44.7416)
  line L85 (23.3486, 45.038) -> (23.3263, 46.027)
  spline S215 degree 3 poles (25.2118, 46.1011) (25.6451, 46.1011) (26.0007, 46.0862) (26.0415, 46.064) knots 0 0 0 0 1 1 1 1
  line L86 (26.2008, 44.6972) -> (27.0453, 44.6935)
  spline S216 degree 3 poles (24.4932, 43.4118) (24.5561, 43.4229) (24.6376, 43.4341) (24.6747, 43.4341) knots 0 0 0 0 1 1 1 1
  spline S217 degree 3 poles (26.6712, 43.5896) (26.6712, 43.4933) (26.6453, 43.3785) (26.6193, 43.3377) knots 0 0 0 0 1 1 1 1
  line L87 (23.3263, 46.027) -> (23.0522, 46.027)
  line L88 (26.2008, 44.6972) -> (27.0453, 44.6935)
  spline S218 degree 3 poles (26.1526, 45.6417) (26.0822, 45.4232) (26.0822, 45.4232) (25.2784, 45.4676) knots 0 0 0 0 1 1 1 1
  spline S219 degree 3 poles (26.0415, 46.064) (26.1489, 46.0084) (26.2045, 45.7936) (26.1526, 45.6417) knots 0 0 0 0 1 1 1 1
  line L89 (23.5708, 43.397) -> (23.8634, 43.397)
  spline S220 degree 3 poles (25.0043, 44.7305) (25.1969, 44.7157) (25.7378, 44.7009) (26.2008, 44.6972) knots 0 0 0 0 1 1 1 1
  spline S221 degree 3 poles (24.0487, 45.1528) (23.9968, 45.7455) (23.9635, 45.9677) (23.9264, 45.9936) knots 0 0 0 0 1 1 1 1
  line L90 (23.5264, 45.4158) -> (23.5264, 44.9342)
  spline S222 degree 3 poles (24.4932, 43.4118) (24.5561, 43.4229) (24.6376, 43.4341) (24.6747, 43.4341) knots 0 0 0 0 1 1 1 1
  spline S223 degree 3 poles (23.8227, 45.0565) (23.9746, 44.5749) (24.1005, 44.2156) (24.1079, 44.2601) knots 0 0 0 0 1 1 1 1
  spline S224 degree 3 poles (23.8227, 45.0565) (23.9746, 44.5749) (24.1005, 44.2156) (24.1079, 44.2601) knots 0 0 0 0 1 1 1 1
  line L91 (27.0453, 44.6935) -> (27.1342, 44.6009)
  spline S225 degree 3 poles (20.463, 42.934) (20.4149, 42.9673) (20.326, 43.0785) (20.2704, 43.1822) knots 0 0 0 0 1 1 1 1
  spline S226 degree 3 poles (25.6192, 44.7416) (25.0377, 44.7527) (24.7932, 44.749) (25.0043, 44.7305) knots 0 0 0 0 1 1 1 1
  line L92 (13.051, 53.0019) -> (13.2066, 53.0834)
  line L93 (26.586, 44.7194) -> (25.6192, 44.7416)
  spline S227 degree 3 poles (22.9004, 43.2896) (22.6707, 43.3118) (22.4744, 43.3229) (22.4633, 43.3155) knots 0 0 0 0 1 1 1 1
  line L94 (19.2999, 43.5822) -> (19.2999, 44.6194)
  spline S228 degree 3 poles (22.7522, 44.4638) (22.7485, 43.9304) (22.7522, 43.4896) (22.7633, 43.4785) knots 0 0 0 0 1 1 1 1
  spline S229 degree 3 poles (24.0487, 45.1528) (23.9968, 45.7455) (23.9635, 45.9677) (23.9264, 45.9936) knots 0 0 0 0 1 1 1 1
  spline S230 degree 3 poles (23.8634, 43.397) (24.0227, 43.397) (24.1524, 43.4118) (24.1524, 43.4303) knots 0 0 0 0 1 1 1 1
  line L95 (26.649, 44.8083) -> (26.586, 44.7194)
  spline S231 degree 3 poles (25.96, 44.0415) (25.2747, 44.0564) (24.8191, 44.0526) (24.8191, 44.0341) knots 0 0 0 0 1 1 1 1
  spline S232 degree 3 poles (22.4633, 43.3155) (22.4559, 43.3044) (22.6114, 43.2525) (22.8078, 43.1933) knots 0 0 0 0 1 1 1 1
  spline S233 degree 3 poles (22.4633, 43.3155) (22.4559, 43.3044) (22.6114, 43.2525) (22.8078, 43.1933) knots 0 0 0 0 1 1 1 1
  spline S234 degree 3 poles (12.2175, 53.0871) (12.1175, 52.8982) (12.1101, 52.4907) (12.2064, 52.2722) knots 0 0 0 0 1 1 1 1
  spline S235 degree 3 poles (23.3375, 43.4229) (23.3412, 43.4415) (23.2115, 43.8971) (23.0522, 44.4416) knots 0 0 0 0 1 1 1 1
  spline S236 degree 3 poles (20.463, 42.934) (20.4149, 42.9673) (20.326, 43.0785) (20.2704, 43.1822) knots 0 0 0 0 1 1 1 1
  spline S237 degree 3 poles (12.0249, 53.0723) (12.099, 53.2945) (12.2842, 53.5057) (12.5176, 53.6316) knots 0 0 0 0 1 1 1 1
  line L96 (19.2999, 44.6194) -> (19.2999, 45.6566)
  spline S238 degree 3 poles (24.245, 44.7676) (24.3672, 43.2933) (24.3524, 43.3822) (24.4932, 43.4118) knots 0 0 0 0 1 1 1 1
  spline S239 degree 3 poles (24.1524, 43.4303) (24.1524, 43.4452) (24.0116, 43.9008) (23.8375, 44.4379) knots 0 0 0 0 1 1 1 1
  spline S240 degree 3 poles (24.245, 44.7676) (24.3672, 43.2933) (24.3524, 43.3822) (24.4932, 43.4118) knots 0 0 0 0 1 1 1 1
  spline S241 degree 3 poles (23.5264, 44.9342) (23.5227, 44.6675) (23.5338, 44.2156) (23.5486, 43.923) knots 0 0 0 0 1 1 1 1
  spline S242 degree 3 poles (24.8191, 44.0341) (24.8191, 43.9934) (25.1451, 43.9637) (25.9637, 43.9304) knots 0 0 0 0 1 1 1 1
  line L97 (19.637, 43.5822) -> (19.2999, 43.5822)
  spline S243 degree 3 poles (20.2704, 43.1822) (20.2148, 43.2896) (20.1259, 43.4229) (20.0704, 43.4785) knots 0 0 0 0 1 1 1 1
  spline S244 degree 3 poles (25.9637, 43.9304) (26.6342, 43.9008) (26.6712, 43.8823) (26.6712, 43.5896) knots 0 0 0 0 1 1 1 1
  spline S245 degree 3 poles (20.2704, 43.1822) (20.2148, 43.2896) (20.1259, 43.4229) (20.0704, 43.4785) knots 0 0 0 0 1 1 1 1
  line L98 (19.2999, 44.6194) -> (19.2999, 45.6566)
  line L99 (19.2999, 45.6566) -> (19.6629, 45.6566)
  spline S246 degree 3 poles (24.6747, 43.4341) (24.7747, 43.4341) (24.7673, 43.6637) (24.6524, 44.2045) knots 0 0 0 0 1 1 1 1
  spline S247 degree 3 poles (24.1524, 43.4303) (24.1524, 43.4452) (24.0116, 43.9008) (23.8375, 44.4379) knots 0 0 0 0 1 1 1 1
  spline S248 degree 3 poles (17.0404, 43.5267) (14.3437, 48.1902) (12.099, 52.0981) (12.0509, 52.2129) knots 0 0 0 0 1 1 1 1
  spline S249 degree 3 poles (12.0249, 53.0723) (12.099, 53.2945) (12.2842, 53.5057) (12.5176, 53.6316) knots 0 0 0 0 1 1 1 1
  spline S250 degree 3 poles (23.3375, 43.4229) (23.3412, 43.4415) (23.2115, 43.8971) (23.0522, 44.4416) knots 0 0 0 0 1 1 1 1
  line L100 (19.2999, 45.6566) -> (19.6629, 45.6566)
  spline S251 degree 3 poles (22.7633, 43.4785) (22.7744, 43.4674) (22.893, 43.4452) (23.0337, 43.4341) knots 0 0 0 0 1 1 1 1
  line L101 (19.637, 43.5822) -> (19.2999, 43.5822)
  line L102 (22.7633, 45.4306) -> (22.7522, 44.4638)
  spline S252 degree 3 poles (25.5562, 45.4047) (26.5416, 45.3713) (26.5749, 45.3676) (26.6416, 45.2861) knots 0 0 0 0 1 1 1 1
  spline S253 degree 3 poles (26.6416, 45.2861) (26.7268, 45.1824) (26.7305, 44.9268) (26.649, 44.8083) knots 0 0 0 0 1 1 1 1
  spline S254 degree 3 poles (20.2593, 45.9603) (20.3111, 46.0455) (20.3852, 46.1122) (20.4593, 46.1344) knots 0 0 0 0 1 1 1 1
  spline S255 degree 3 poles (21.9373, 42.6562) (21.0483, 42.7969) (20.5223, 42.8932) (20.463, 42.934) knots 0 0 0 0 1 1 1 1
  spline S256 degree 3 poles (12.0509, 52.2129) (11.9508, 52.4574) (11.9397, 52.8241) (12.0249, 53.0723) knots 0 0 0 0 1 1 1 1
  spline S257 degree 3 poles (24.8191, 44.0341) (24.8191, 43.9934) (25.1451, 43.9637) (25.9637, 43.9304) knots 0 0 0 0 1 1 1 1
  line L103 (27.0453, 44.6935) -> (27.1342, 44.6009)
  spline S258 degree 3 poles (25.0043, 44.7305) (25.1969, 44.7157) (25.7378, 44.7009) (26.2008, 44.6972) knots 0 0 0 0 1 1 1 1
  line L104 (19.2999, 43.5822) -> (19.2999, 44.6194)
  spline S259 degree 3 poles (22.5411, 43.7674) (22.5522, 43.7674) (22.5596, 44.2749) (22.5596, 44.8972) knots 0 0 0 0 1 1 1 1
  spline S260 degree 3 poles (24.6747, 43.4341) (24.7747, 43.4341) (24.7673, 43.6637) (24.6524, 44.2045) knots 0 0 0 0 1 1 1 1
  line L105 (22.7633, 45.4306) -> (22.7522, 44.4638)
  line L106 (22.5596, 44.8972) -> (22.5596, 46.027)
  spline S261 degree 3 poles (21.9373, 42.6562) (21.0483, 42.7969) (20.5223, 42.8932) (20.463, 42.934) knots 0 0 0 0 1 1 1 1
  spline S262 degree 3 poles (26.6193, 43.3377) (26.5638, 43.2637) (26.5379, 43.26) (24.9414, 43.2563) knots 0 0 0 0 1 1 1 1
  spline S263 degree 3 poles (22.5411, 43.7674) (22.5522, 43.7674) (22.5596, 44.2749) (22.5596, 44.8972) knots 0 0 0 0 1 1 1 1
  spline S264 degree 3 poles (20.2593, 45.9603) (20.3111, 46.0455) (20.3852, 46.1122) (20.4593, 46.1344) knots 0 0 0 0 1 1 1 1
  spline S265 degree 3 poles (27.7602, 44.3156) (30.3198, 48.6643) (32.4127, 52.224) (32.4127, 52.2352) knots 0 0 0 0 1 1 1 1
  line L107 (23.0004, 53.0945) -> (32.7942, 53.1019)
  spline S266 degree 3 poles (28.8307, 43.6267) (31.557, 48.3198) (33.8239, 52.2463) (33.861, 52.3574) knots 0 0 0 0 1 1 1 1
  spline S267 degree 3 poles (33.2831, 53.5724) (33.109, 53.6353) (32.5423, 53.639) (23.0411, 53.639) knots 0 0 0 0 1 1 1 1
  spline S268 degree 3 poles (22.7929, 34.6144) (22.9485, 34.5774) (23.1967, 34.607) (23.3856, 34.6885) knots 0 0 0 0 1 1 1 1
  spline S269 degree 3 poles (24.1079, 44.2601) (24.1116, 44.3045) (24.0857, 44.7046) (24.0487, 45.1528) knots 0 0 0 0 1 1 1 1
  line L108 (23.5708, 43.397) -> (23.8634, 43.397)
  line L109 (23.3486, 45.038) -> (23.3263, 46.027)
  spline S270 degree 3 poles (19.6629, 45.6566) (20.0667, 45.6566) (20.0815, 45.664) (20.2593, 45.9603) knots 0 0 0 0 1 1 1 1
  line L110 (21.8558, 49.031) -> (21.8558, 50.4942)
  spline S271 degree 3 poles (23.5264, 44.9342) (23.5227, 44.6675) (23.5338, 44.2156) (23.5486, 43.923) knots 0 0 0 0 1 1 1 1
  spline S272 degree 3 poles (22.2632, 46.027) (22.0336, 46.027) (21.9669, 46.0159) (21.9669, 45.9751) knots 0 0 0 0 1 1 1 1
  spline S273 degree 3 poles (25.2784, 45.4676) (24.6154, 45.5047) (24.4783, 45.501) (24.5265, 45.4565) knots 0 0 0 0 1 1 1 1
  spline S274 degree 3 poles (22.2632, 46.027) (22.0336, 46.027) (21.9669, 46.0159) (21.9669, 45.9751) knots 0 0 0 0 1 1 1 1
  spline S275 degree 3 poles (12.7213, 52.3463) (12.6695, 52.6315) (12.7843, 52.8575) (13.051, 53.0019) knots 0 0 0 0 1 1 1 1
  spline S276 degree 3 poles (20.0704, 43.4785) (19.9778, 43.5785) (19.9555, 43.5822) (19.637, 43.5822) knots 0 0 0 0 1 1 1 1
  spline S277 degree 3 poles (27.1342, 44.6009) (27.2453, 44.4934) (27.2602, 44.2416) (27.1639, 44.1045) knots 0 0 0 0 1 1 1 1
  line L111 (22.5596, 46.027) -> (22.2632, 46.027)
  spline S278 degree 3 poles (22.9004, 43.2896) (22.6707, 43.3118) (22.4744, 43.3229) (22.4633, 43.3155) knots 0 0 0 0 1 1 1 1
  spline S279 degree 3 poles (27.1342, 44.6009) (27.2453, 44.4934) (27.2602, 44.2416) (27.1639, 44.1045) knots 0 0 0 0 1 1 1 1
  spline S280 degree 3 poles (12.2175, 53.0871) (12.1175, 52.8982) (12.1101, 52.4907) (12.2064, 52.2722) knots 0 0 0 0 1 1 1 1
  line L112 (22.5596, 44.8972) -> (22.5596, 46.027)
  spline S281 degree 3 poles (21.9669, 45.9751) (21.9669, 45.7269) (22.4781, 43.7674) (22.5411, 43.7674) knots 0 0 0 0 1 1 1 1
  spline S282 degree 3 poles (17.0404, 43.5267) (14.3437, 48.1902) (12.099, 52.0981) (12.0509, 52.2129) knots 0 0 0 0 1 1 1 1
  line L113 (21.8558, 50.4942) -> (21.8558, 51.9536)
  spline S283 degree 3 poles (12.0509, 52.2129) (11.9508, 52.4574) (11.9397, 52.8241) (12.0249, 53.0723) knots 0 0 0 0 1 1 1 1
  spline S284 degree 3 poles (25.2784, 45.4676) (24.6154, 45.5047) (24.4783, 45.501) (24.5265, 45.4565) knots 0 0 0 0 1 1 1 1
  spline S285 degree 3 poles (12.7954, 53.5724) (12.562, 53.4909) (12.3213, 53.2908) (12.2175, 53.0871) knots 0 0 0 0 1 1 1 1
  line L114 (21.8558, 51.9536) -> (22.7077, 51.9536)
  line L115 (22.6929, 47.9568) -> (21.8558, 49.031)
  line L116 (21.8558, 49.031) -> (21.8558, 50.4942)
  spline S286 degree 3 poles (24.182, 46.1381) (24.3302, 46.1196) (24.7969, 46.1011) (25.2118, 46.1011) knots 0 0 0 0 1 1 1 1
  line L117 (21.8558, 50.4942) -> (21.8558, 51.9536)
  spline S287 degree 3 poles (20.0704, 43.4785) (19.9778, 43.5785) (19.9555, 43.5822) (19.637, 43.5822) knots 0 0 0 0 1 1 1 1
  line L118 (22.5596, 46.027) -> (22.2632, 46.027)
  spline S288 degree 3 poles (19.6629, 45.6566) (20.0667, 45.6566) (20.0815, 45.664) (20.2593, 45.9603) knots 0 0 0 0 1 1 1 1
  spline S289 degree 3 poles (28.8307, 43.6267) (31.557, 48.3198) (33.8239, 52.2463) (33.861, 52.3574) knots 0 0 0 0 1 1 1 1
  spline S290 degree 3 poles (33.2868, 52.2389) (33.2609, 52.1722) (31.068, 48.3865) (28.4159, 43.823) knots 0 0 0 0 1 1 1 1
  spline S291 degree 3 poles (22.9633, 35.1367) (22.9337, 35.1367) (22.8448, 35.1701) (22.7633, 35.2071) knots 0 0 0 0 1 1 1 1
  spline S292 degree 3 poles (23.0411, 52.25) (17.8849, 52.25) (13.6696, 52.2389) (13.6696, 52.2277) knots 0 0 0 0 1 1 1 1
  spline S293 degree 3 poles (20.4593, 46.1344) (20.663, 46.2011) (23.7079, 46.2048) (24.182, 46.1381) knots 0 0 0 0 1 1 1 1
  spline S294 degree 3 poles (22.2151, 34.9997) (22.3521, 34.8293) (22.604, 34.6626) (22.7929, 34.6144) knots 0 0 0 0 1 1 1 1
  spline S295 degree 3 poles (22.7633, 35.2071) (22.6818, 35.2441) (22.5781, 35.3145) (22.5336, 35.3627) knots 0 0 0 0 1 1 1 1
  spline S296 degree 3 poles (22.8078, 43.1933) (23.2226, 43.0785) (23.33, 43.0007) (23.4486, 42.7229) knots 0 0 0 0 1 1 1 1
  line L119 (13.2066, 53.0834) -> (23.0004, 53.0945)
  spline S297 degree 3 poles (12.7213, 52.3463) (12.6695, 52.6315) (12.7843, 52.8575) (13.051, 53.0019) knots 0 0 0 0 1 1 1 1
  spline S298 degree 3 poles (23.5597, 49.4163) (23.5597, 48.0198) (23.5523, 46.8789) (23.5449, 46.8789) knots 0 0 0 0 1 1 1 1
  spline S299 degree 3 poles (22.7633, 35.2071) (22.6818, 35.2441) (22.5781, 35.3145) (22.5336, 35.3627) knots 0 0 0 0 1 1 1 1
  spline S300 degree 3 poles (23.7079, 34.9256) (23.8264, 35.0515) (25.2303, 37.437) (28.8307, 43.6267) knots 0 0 0 0 1 1 1 1
  line L120 (22.7077, 51.9536) -> (23.5597, 51.9536)
  spline S301 degree 3 poles (23.4041, 42.4376) (23.356, 42.4413) (22.6966, 42.5376) (21.9373, 42.6562) knots 0 0 0 0 1 1 1 1
  spline S302 degree 3 poles (24.182, 46.1381) (24.3302, 46.1196) (24.7969, 46.1011) (25.2118, 46.1011) knots 0 0 0 0 1 1 1 1
  spline S303 degree 3 poles (23.0337, 43.4341) (23.1708, 43.4192) (23.293, 43.4044) (23.3115, 43.4007) knots 0 0 0 0 1 1 1 1
  spline S304 degree 3 poles (24.5265, 45.4565) (24.5339, 45.4491) (24.9969, 45.4269) (25.5562, 45.4047) knots 0 0 0 0 1 1 1 1
  spline S305 degree 3 poles (22.8078, 43.1933) (23.2226, 43.0785) (23.33, 43.0007) (23.4486, 42.7229) knots 0 0 0 0 1 1 1 1
  spline S306 degree 3 poles (22.5966, 34.4959) (22.4892, 34.5366) (22.3484, 34.6404) (22.1855, 34.7996) knots 0 0 0 0 1 1 1 1
  spline S307 degree 3 poles (22.7818, 45.9973) (22.7781, 45.9529) (23.3523, 44.0304) (23.3634, 44.0415) knots 0 0 0 0 1 1 1 1
  spline S308 degree 3 poles (12.5176, 53.6316) (12.9213, 53.8539) (12.3139, 53.8428) (23.0448, 53.8428) knots 0 0 0 0 1 1 1 1